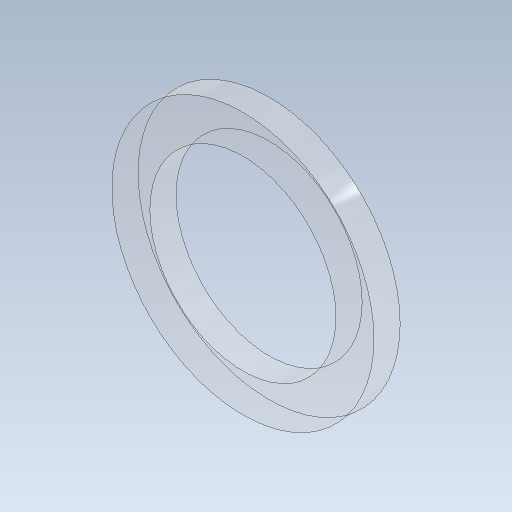
# Autodesk Inventor part: 原動節2補助パーツ
Saved by Autodesk Inventor 2020.4 (Build 244396000, 396)
## iProperties
Created: 2021-05-01
Part Number: 原動節2補助パーツ
Material: ポリカーボネート、クリア
Document SubType Name: Modeling
Designer: happy
Density: 1.2 g/cm^3
Appearance: ポリカーボネート - クリア
Mass: 0.3739 g
Surface Area: 5.26468 cm^2
Volume: 0.311583 cm^3
Author: happy
Autodesk Inventor part; units mm, degrees
ref_plane "YZ Plane" through (0, 0, 0) normal (1, 0, 0) x (0, 1, 0)
ref_plane "XZ Plane" through (0, 0, 0) normal (0, 1, 0) x (-1, 0, 0)
ref_plane "XY Plane" through (0, 0, 0) normal (0, 0, 1) x (1, 0, 0)
sketch "スケッチ1" plane through (0, 0, 0) normal (0, 0, 1) x (1, 0, 0)
  circle A0 centre (0, 0) radius 7.1
  circle A1 centre (0, 0) radius 10
  dimension "d0" = 14.2
  dimension "d1" = 20
  constraints: 2 centre point, 2 coincident
  measures "d0" diameter of A0
  measures "d1" diameter of A1
extrude "押し出し1" add sketch "スケッチ1" along normal blind 2
